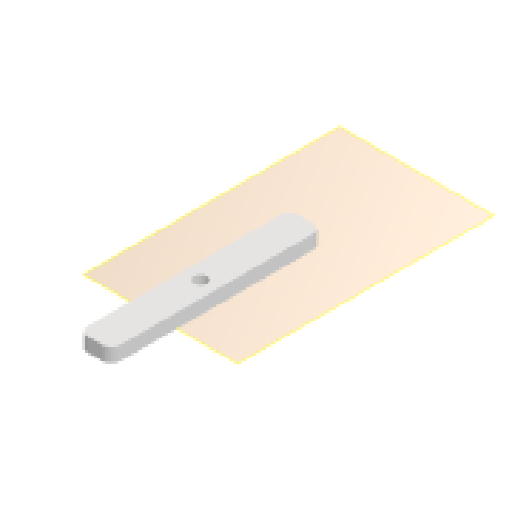
# Autodesk Inventor part: 20_Cube_4_insert_xy_levelarm_2
Saved by Autodesk Inventor 2025.1 (Build 291241020, 241B)
## iProperties
Created: 2024-10-07
Part Number: 20_Cube_4_insert_xy_levelarm_2
Material: Generic
Document SubType Name: Modeling
Designer: diederichbenedict
Density: 1 g/cm^3
Appearance: Default
Author: diederichbenedict
Autodesk Inventor part; units mm, degrees
ref_plane "YZ Plane" through (0, 0, 0) normal (1, 0, 0) x (0, 1, 0)
ref_plane "XZ Plane" through (0, 0, 0) normal (0, 1, 0) x (-1, 0, 0)
ref_plane "XY Plane" through (0, 0, 0) normal (0, 0, 1) x (1, 0, 0)
ref_plane "Work Plane1" through (0, 0, 0) normal (0, 0, 1) x (1, 0, 0)
sketch "Sketch1" plane through (0, 0, 0) normal (0, 0, 1) x (1, 0, 0)
  circle A0 centre (0, -18.9) radius 1.4 projected
  line L0 (1.5, -41.4) -> (-1.5, -41.4)
  line L1 (-3.5, -39.4) -> (-3.5, 1.6)
  line L2 (-1.5, 3.6) -> (1.5, 3.6)
  line L3 (3.5, 1.6) -> (3.5, -39.4)
  line L4 (3.5, -41.4) -> (-3.5, 3.6) construction
  line L5 (-3.5, -41.4) -> (3.5, 3.6) construction
  arc A1 (-3.5, -39.4) -> (-1.5, -41.4) centre (-1.5, -39.4) ccw
  arc A2 (1.5, -41.4) -> (3.5, -39.4) centre (1.5, -39.4) ccw
  arc A3 (3.5, 1.6) -> (1.5, 3.6) centre (1.5, 1.6) ccw
  arc A4 (-1.5, 3.6) -> (-3.5, 1.6) centre (-1.5, 1.6) ccw
  point P0 (0, 0)
  dimension "d0" = 7
  dimension "d1" = 45
  dimension "d2" = 2
  constraints: 12 end point, 8 point on circle, 8 point on line, 8 tangent, 4 centre point, 3 equal radius, 2 midpoint, 2 parallel, 1 horizontal, 1 perpendicular
  measures "d0" distance of L4.end L5.end
  measures "d1" distance of L5.start L4.end
  measures "d2" radius of A1
extrude "Extrusion1" add sketch "Sketch1" along normal blind 3
body "Solid1"
